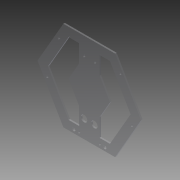
# Autodesk Inventor part: Top Plate
Saved by Autodesk Inventor 2015 (Build 190159000, 159)
## iProperties
Created: 2016-02-26
Part Number: Top Plate
Material: Polycarbonate, Clear
Document SubType Name: Modeling
Designer: James Yelland
Density: 1.2 g/cm^3
Appearance: Polycarbonate - Clear
Author: James Yelland
Autodesk Inventor part; units mm, degrees
ref_plane "YZ Plane" through (0, 0, 0) normal (1, 0, 0) x (0, 1, 0)
ref_plane "XZ Plane" through (0, 0, 0) normal (0, 1, 0) x (-1, 0, 0)
ref_plane "XY Plane" through (0, 0, 0) normal (0, 0, 1) x (1, 0, 0)
sketch "Sketch1" plane through (0, 0, 0) normal (0, 1, 0) x (-1, 0, 0)
  line L0 (-50, 86.6025) -> (-100, 0)
  line L1 (-100, 0) -> (-50, -86.6025)
  line L2 (-50, -86.6025) -> (50, -86.6025)
  line L3 (50, -86.6025) -> (100, 0)
  line L4 (100, 0) -> (50, 86.6025)
  line L5 (50, 86.6025) -> (-50, 86.6025)
  circle A0 centre (20, -80.1075) radius 1.6
  circle A1 centre (-20, -80.1075) radius 1.6
  line L6 (-80, 0) -> (-40, 69.282)
  line L7 (-40, 69.282) -> (-20, 69.282)
  line L8 (-80, 0) -> (-40, -69.282)
  line L9 (-40, -69.282) -> (-20, -69.282)
  line L10 (20, -69.282) -> (40, -69.282)
  line L11 (40, -69.282) -> (80, 0)
  line L12 (80, 0) -> (40, 69.282)
  line L13 (40, 69.282) -> (20, 69.282)
  line L14 (-20, 69.282) -> (-20, 34.641)
  line L15 (20, 69.282) -> (20, 34.641)
  line L16 (20, -69.282) -> (20, -34.641)
  line L17 (-20, -69.282) -> (-20, -34.641)
  line L18 (-20, -34.641) -> (-40, 0)
  line L19 (-40, 0) -> (-20, 34.641)
  line L20 (20, 34.641) -> (40, 0)
  line L21 (40, 0) -> (20, -34.641)
  circle A2 centre (-10, -51.9615) radius 6.25
  circle A3 centre (10, -51.9615) radius 6.25
  circle A4 centre (-10.5, 51.9615) radius 1.65
  circle A5 centre (10.5, 51.9615) radius 1.6
  circle A6 centre (-59.3781, 57.3685) radius 1.6
  circle A7 centre (-81.8748, -18.4029) radius 1.6
  circle A8 centre (59.3781, 57.3685) radius 1.6
  circle A9 centre (81.8767, -18.3996) radius 1.6
  circle A10 centre (-30, -80.1075) radius 3
  circle A11 centre (30, -80.1075) radius 3
  dimension "d12" = 6
  dimension "d13" = 6
  constraints: 44 end point, 12 centre point
  measures "d12" diameter of A10
  measures "d13" diameter of A11
extrude "Extrusion1" add sketch "Sketch1" along normal blind 3
sketch "Sketch6" plane through (0, 3, 0) normal (0, 1, 0) x (1, 0, 0)
  line L0 (0, 0) -> (0, -34.641)
  line L1 (0, 0) -> (-40, 0)
  line L2 (17.5, -17.5) -> (-17.5, -17.5) construction
  line L3 (-17.5, -17.5) -> (-17.5, 17.5) construction
  line L4 (-17.5, 17.5) -> (17.5, 17.5) construction
  line L5 (17.5, 17.5) -> (17.5, -17.5) construction
  dimension "d58" = 35
  dimension "d70" = 17.5
  dimension "d72" = 17.5
  constraints: 4 end point, 1 horizontal, 1 vertical, 2 other
  measures "d58" distance of L2.start L2.end
  measures "d70" distance between parallel lines of L3 L0
  measures "d72" distance between parallel lines of L2 L1
decal "Decal1"
body "Solid1"
